Autodesk Inventor part; units mm, degrees
(part 2 of 2)
  point P85 (-11.3848, -38.0261)
  point P86 (-11.3848, -35.4744)
  point P87 (-13.8848, -35.4744)
  point P88 (-13.8848, -38.0261)
  dimension "d0" = 43
  dimension "d1" = 85
  dimension "d6" = 2.5
  dimension "d7" = 2.5
  dimension "d8" = 2.5
  dimension "d9" = 2.5
  dimension "d10" = 2.5
  dimension "d11" = 2.5
  dimension "d12" = 2.5
  dimension "d13" = 2.5
  dimension "d14" = 1
  dimension "d20" = 1
  dimension "d21" = 1
  dimension "d22" = 1
  dimension "d23" = 2.5
  dimension "d24" = 2.5
  dimension "d25" = 2.5
  dimension "d26" = 1.8202
  dimension "d27" = 1.8202
  dimension "d28" = 2.1798
  dimension "d29" = 2.1798
  constraints: 1228 symmetric about line, 650 end point, 592 centre point, 138 point on line, 11 horizontal, 10 midpoint, 6 perpendicular, 2 vertical, 1 parallel, 597 other
  measures "d0" distance of L1.end L2.end
  measures "d1" distance of L0.end L1.end
  measures "d6" distance between parallel lines of L5 L6
  measures "d7" distance between parallel lines of L4 L5
  measures "d8" distance between parallel lines of L8 L4
  measures "d9" distance between parallel lines of L13 L8
  measures "d10" distance between parallel lines of L9 L13
  measures "d11" distance between parallel lines of L12 L9
  measures "d12" distance between parallel lines of L11 L12
  measures "d13" distance between parallel lines of L10 L11
  measures "d14" diameter of A0
  measures "d20" diameter of A2
  measures "d21" diameter of A4
  measures "d22" diameter of A6
  measures "d23" horizontal distance of A2.centre A1.centre
  measures "d24" distance of A4.centre A3.centre
  measures "d25" distance of A6.centre A5.centre
  measures "d26" distance from line of L14 A7.centre
  measures "d27" distance from line of L14 A14.centre
  measures "d28" distance from line of L1 A8.centre
extrude "Extrusion1" add sketch "Sketch1" against normal blind 0.001 contours L0 L14 L2 L3 | L0 L1 L2 L14 | A0 | A1 | A2 | A3 | A4 | A5 | A6 | A7 | A8 | A9 | A10 | A11 | A12 | A13 | A14 | A15 | A16 | A17 | A18 | A19 | A20 | A21 | A22 | A23 | A24 | A25 | A26 | A27 | A28 | A29 | A30 | A31 | A32 | A33 | A34 | A35 | A36 | A37 | A38 | A39 | A40 | A41 | A42 | A43 | A44 | A45 | A46 | A47 | A48 | A49 | A50 | A51 | A52 | A53 | A54 | A55 | A56 | A57 | A58 | A59 | A60 | A61 | A62 | A63 | A64 | A65 | A66 | A67 | A68 | A69 | A70 | A71 | A72 | A73 | A74 | A75 | A76 | A77 | A78 | A79 | A80 | A81 | A82 | A83 | A84 | A85 | A86 | A87 | A88 | A89 | A90 | A91 | A92 | A93 | A94 | A95 | A96 | A97 | A98 | A99 | A100 | A101 | A102 | A103 | A104 | A105 | A106 | A107 | A108 | A109 | A110 | A111 | A112 | A113 | A114 | A115 | A116 | A117 | A118 | A119 | A120 | A121 | A122 | A123 | A124 | A125 | A126 | A127 | A128 | A129 | A130 | A131 | A132 | A133 | A134 | A135 | A136 | A137 | A138 | A139 | A140 | A141 | A142 | A143 | A144 | A145 | A146 | A147 | A148 | A149 | A150 | A151 | A152 | A153 | A154 | A155 | A156 | A157 | A158 | A159 | A160 | A161 | A162 | A163 | A164 | A165 | A166 | A167 | A168 | A169 | A170 | A171 | A172 | A173 | A174 | A175 | A176 | A177 | A178 | A179 | A180 | A181 | A182 | A183 | A184 | A185 | A186 | A187 | A188 | A189 | A190 | A191 | A192 | A193 | A194 | A195 | A196 | A197 | A198 | A199 | A200 | A201 | A202 | A203 | A204 | A205 | A206 | A207 | A208 | A209 | A210 | A211 | A212 | A213 | A214 | A215 | A216 | A217 | A218 | A219 | A220 | A221 | A222 | A223 | A224 | A225 | A226 | A227 | A228 | A229 | A230 | A231 | A232 | A233 | A234 | A235 | A236 | A237 | A238 | A239 | A240 | A241 | A242 | A243 | A244 | A245 | A246 | A247 | A248 | A249 | A250 | A251 | A252 | A253 | A254 | A255 | A256 | A257 | A258 | A259 | A260 | A261 | A262 | A263 | A264 | A265 | A266 | A267 | A268 | A269 | A270 | A271 | A272 | A273 | A274 | A275 | A276 | A277 | A278 | A279 | A280 | A281 | A282 | A283 | A284 | A285 | A286 | A287 | A288 | A289 | A290 | A296 | A306 | A309 | A310 | A311 | A312 | A313 | A314 | A315 | A316 | A317 | A318 | A319 | A320 | A321 | A322 | A323 | A324 | A325 | A326 | A327 | A328 | A329 | A330 | A331 | A332 | A333 | A334 | A335 | A336 | A337 | A338 | A339 | A340 | A341 | A342 | A343 | A344 | A345 | A346 | A347 | A348 | A349 | A350 | A351 | A352 | A353 | A354 | A355 | A356 | A357 | A358 | A359 | A360 | A361 | A362 | A363 | A364 | A365 | A366 | A367 | A368 | A369 | A370 | A371 | A372 | A373 | A374 | A375 | A376 | A377 | A378 | A379 | A380 | A381 | A382 | A383 | A384 | A385 | A386 | A387 | A388 | A389 | A390 | A391 | A392 | A393 | A394 | A395 | A396 | A397 | A398 | A399 | A400 | A401 | A402 | A403 | A404 | A405 | A406 | A407 | A408 | A409 | A410 | A411 | A412 | A413 | A414 | A415 | A416 | A417 | A418 | A419 | A420 | A421 | A422 | A423 | A424 | A425 | A426 | A427 | A428 | A429 | A430 | A431 | A433 | A435 | A438 | A439 | A440 | A441 | A443 | A445 | A446 | A447 | A448 | A449 | A450 | A451 | A461 | A462 | A463 | A464 | A465 | A466 | A467 | A468 | A469 | A470 | A471 | A473 | A474 | A475 | A476 | A477 | A478 | A479 | A480 | A481 | A482 | A483 | A484 | A485 | A486 | A487 | A488 | A489 | A490 | A491 | A496 | A497 | A498 | A499 | A500 | A501 | A502 | A503 | A504 | A505 | A509 | A510 | A512 | A513 | A515 | A516 | A517 | A518 | A522 | A523 | A524 | A525 | A526 | A527 | A528 | A529 | A531 | A532 | A534 | A535 | A536 | A537 | A538 | A539 | A540 | A543 | A545 | A546 | A547 | A548 | A549 | A550 | A551 | A555 | A557 | A558 | A559 | A561 | A562 | A563 | A565 | A568 | A569 | A571 | A572 | A574 | A575 | A576 | A577 | A581 | A583 | A584 | A585 | A587 | A588 | A589 | A590 | A591
extrude "Extrusion2" add sketch "Sketch1" along normal blind 2
body "Solid1"
